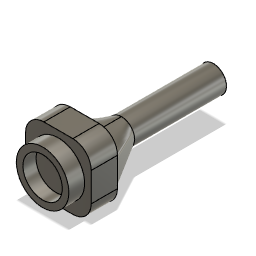
Axial+rotator+left (Autodesk Fusion 360 design; units mm, degrees)
Autodesk Fusion 360 part; units mm, degrees
note: some values were not read from the file. Set by a fixed rule: which sketch regions a step uses.
sketch "Sketch1" plane through (0, 0, 0) normal (0, 0, 1) x (1, 0, 0)
  circle A0 centre (0, 0) radius 7.5
  line L0 (-5.5, 12.5) -> (5.5, 12.5)
  line L1 (12.5, 5.5) -> (12.5, -5.5)
  line L2 (5.5, -12.5) -> (-5.5, -12.5)
  line L3 (-12.5, -5.5) -> (-12.5, 5.5)
  circle A1 centre (0, 0) radius 10
  arc A2 (-5.5, 12.5) -> (-12.5, 5.5) centre (-5.5, 5.5) ccw
  arc A3 (12.5, 5.5) -> (5.5, 12.5) centre (5.5, 5.5) ccw
  arc A4 (5.5, -12.5) -> (12.5, -5.5) centre (5.5, -5.5) ccw
  arc A5 (-12.5, -5.5) -> (-5.5, -12.5) centre (-5.5, -5.5) ccw
  line L4 (-10.4497, 10.4497) -> (10.4497, -10.4497)
  line L5 (10.4497, 10.4497) -> (0, 0)
  point P0 (-12.5, 12.5)
  dimension "d1" = 15
  dimension "d2" = 20
  dimension "d5" = 7
  constraint coincident A0.centre A1.centre
  constraint horizontal L0
  constraint vertical L1
  constraint horizontal L2
  constraint vertical L3
  constraint coincident P0 L3
  constraint coincident P0 L0
  constraint tangent L3 A2
  constraint tangent L0 A2
  constraint tangent L0 A3
  constraint tangent L1 A3
  constraint equal A2 A3
  constraint tangent L1 A4
  constraint tangent L2 A4
  constraint equal A2 A4
  constraint tangent L2 A5
  constraint tangent L3 A5
  constraint equal A2 A5
  constraint midpoint A2 L4.start
  constraint midpoint A4 L4.end
  constraint midpoint A3 L5.start
  constraint midpoint L4 A0.centre
  constraint perpendicular L4 L5
  measures "d1" diameter of A0
  measures "d2" diameter of A1
  measures "d5" radius of A2
extrude "Extrude1" add sketch "Sketch1" along normal blind 10 contours L1 A1 A3 A4 L4 L5 | L0 A1 A2 A3 L4 L5 | L2 L3 A1 A2 A4 A5 L4 makes body 1
extrude "Extrude2" add sketch "Sketch1" along normal blind 16 contours A0 A1 L4 L5 | A0 A1 L4 L5 | A0 A1 L4 bodies 1
extrude "Extrude3" add sketch "Sketch1" along normal blind 11 contours A0 L4 L5 | A0 L4 L5 | A0 L4 bodies 1
sketch "Sketch2" plane through (0, 0, 0) normal (1, 0, 0) x (0, 0, -1)
  line L0 (14.0161, 0) -> (49.0161, 0)
  line L1 (49.0161, 0) -> (49.0161, 5)
  line L2 (49.0161, 5) -> (14.0161, 5)
  line L3 (14.0161, 5) -> (14.0161, 0)
  dimension "d12" = 35
  dimension "d13" = 5
  constraint horizontal L0
  constraint vertical L1
  constraint horizontal L2
  constraint vertical L3
  measures "d12" distance of L0.start L0.end
  measures "d13" distance of L0.start L2.end
revolve "Revolve1" add sketch "Sketch2" angle 360 about axis through (0, 0, -14.0161) along (0, 0, -1) separate body makes body 2
sketch "Sketch3" plane through (0, 0, 0) normal (0, 0, -1) x (-1, 0, 0)
  arc A0 (12.5, 5.5) -> (5.5, 12.5) centre (5.5, 5.5) ccw
  line L0 (5.5, 12.5) -> (-5.5, 12.5)
  arc A1 (-5.5, 12.5) -> (-12.5, 5.5) centre (-5.5, 5.5) ccw
  line L1 (-12.5, 5.5) -> (-12.5, -5.5)
  arc A2 (-12.5, -5.5) -> (-5.5, -12.5) centre (-5.5, -5.5) ccw
  line L2 (-5.5, -12.5) -> (5.5, -12.5)
  arc A3 (5.5, -12.5) -> (12.5, -5.5) centre (5.5, -5.5) ccw
  line L3 (12.5, -5.5) -> (12.5, 5.5)
  line L4 (-11.5, 5) -> (11.5, 5)
  line L5 (11.5, -5) -> (-11.5, -5)
  line L6 (-12.5, -4) -> (-12.5, 4)
  arc A4 (-11.5, 5) -> (-12.5, 4) centre (-11.5, 4) ccw
  arc A5 (-12.5, -4) -> (-11.5, -5) centre (-11.5, -4) ccw
  line L7 (-12.5, 0) -> (17.5, 0) construction
  line L8 (12.5, 4) -> (12.5, -4)
  arc A6 (12.5, 4) -> (11.5, 5) centre (11.5, 4) ccw
  arc A7 (11.5, -5) -> (12.5, -4) centre (11.5, -4) ccw
  point P0 (-12.5, 5)
  point P1 (-12.5, -5)
  dimension "d15" = 10
  dimension "d16" = 1
  dimension "d17" = 1
  constraint horizontal L4
  constraint horizontal L5
  constraint vertical L6
  constraint coincident L1 P0
  constraint coincident P0 L6
  constraint coincident P0 L4
  constraint tangent L6 A4
  constraint tangent L4 A4
  constraint coincident P1 L5
  constraint coincident P1 L6
  constraint tangent L5 A5
  constraint tangent L6 A5
  constraint equal A4 A5
  constraint midpoint L6 L7.start
  constraint coincident origin L7
  constraint tangent L4 A6
  constraint tangent L8 A6
  constraint tangent L5 A7
  constraint tangent L8 A7
  constraint equal A6 A7
  measures "d15" distance of P0 P1
  measures "d16" radius of A4
  measures "d17" radius of A6
loft "Loft1" add profiles "Sketch3" section 1 contours L1 L3 L4 L5 L6 A4 A5 L8 A6 A7 section 2 face at (-1.5459, -1.0946, -14.0161) on bodies 2 bodies 2 1
